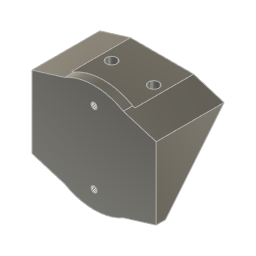
mount (Autodesk Fusion 360 design; units mm, degrees)
Autodesk Fusion 360 part; units mm, degrees
sketch "Sketch1" plane through (0, 0, 0) normal (0, 1, 0) x (1, 0, 0)
  circle A0 centre (0, 0) radius 1.4
  circle A1 centre (0, -30.9) radius 1.4
  line L0 (0, -30.9) -> (0, 0) construction
  line L1 (-26.5, -15.45) -> (26.5, -15.45) construction
  line L2 (26.5, -0.05) -> (-26.5, -0.05)
  line L3 (-26.5, -0.05) -> (-26.5, -30.85)
  line L4 (-26.5, -30.85) -> (26.5, -30.85)
  line L5 (26.5, -30.85) -> (26.5, -0.05)
  line L6 (26.5, -0.05) -> (-26.5, -30.85) construction
  line L7 (-26.5, -0.05) -> (26.5, -30.85) construction
  line L8 (0, -38.45) -> (0, 7.55) construction
  line L9 (-26.5, -30.85) -> (-12.5, -35.15)
  line L10 (-12.5, -35.15) -> (0, -35.15)
  line L11 (26.5, -30.85) -> (12.5, -35.15)
  arc A2 (-12.5, -35.15) -> (12.5, -35.15) centre (0, -13.1258) ccw
  line L12 (-26.5, -0.05) -> (-12.5, 4.25)
  arc A3 (12.5, 4.25) -> (-12.5, 4.25) centre (0, -17.7742) ccw
  line L13 (26.5, -0.05) -> (12.5, 4.25)
  point P0 (0, -15.45)
  point P1 (0, -15.45)
  point P2 (0, -15.45)
  point P3 (0, -15.45)
  dimension "d1" = 2.8
  dimension "d2" = 2.8
  dimension "d3" = 30.9
  dimension "d4" = 53
  dimension "d5" = 53
  dimension "d6" = 30.8
  dimension "d7" = 14
  dimension "d8" = 19.7
  dimension "d9" = 46
  constraint coincident A0.centre L0.end
  constraint coincident A1.centre L0.start
  constraint vertical L0
  constraint horizontal L1
  constraint midpoint L1 P3
  constraint midpoint L0 P3
  constraint coincident P3 P2
  constraint horizontal L2
  constraint perpendicular L2 L3
  constraint parallel L2 L4
  constraint parallel L3 L5
  constraint coincident L6 P3
  constraint coincident L7 P3
  constraint perpendicular L1 L8
  constraint midpoint L8 P3
  constraint coincident L8 L10.end
  constraint perpendicular L8 L10
  constraint symmetric L3.end L8 L4.end
  constraint symmetric L8 L9.end L11.end
  constraint coincident L8.start A2
  constraint symmetric L1 L3.end L2.end
  constraint symmetric L1 L9.end L12.end
  constraint symmetric L1 L4.end L2.start
  constraint symmetric L1 L11.end A3.start
  constraint symmetric L1 A2 A3
  measures "d1" diameter of A1
  measures "d2" diameter of A0
  measures "d3" distance of A0.centre A1.centre
  measures "d4" distance of L1.start L1.end
  measures "d5" distance of L3.end L4.end
  measures "d6" distance of L2.end L3.end
  measures "d7" horizontal distance of L3.end L9.end
  measures "d8" distance of L1 L9.end
  measures "d9" distance of L8.start L8.end
extrude "Extrude1" add sketch "Sketch1" along normal blind 4
hole "Hole1" at (0, 0, 30.9) at (0, 0, 0) direction (0, 1, 0) diameter 2.529 end through all
thread "Thread1" "ISO Metric profile 3.0 M3x0.5 6H"
sketch "Sketch2" plane through (0, 4, 0) normal (0, 1, 0) x (-1, 0, 0)
  circle A0 centre (0, 30.9) radius 1.2645
  circle A1 centre (0, 0) radius 1.2645
  line L0 (-26.5, 30.85) -> (-26.5, 0.05)
  line L1 (-26.5, 0.05) -> (-12.5, -4.25)
  arc A2 (-12.5, -4.25) -> (12.5, -4.25) centre (0, 17.7742) ccw
  line L2 (12.5, -4.25) -> (26.5, 0.05)
  line L3 (26.5, 0.05) -> (26.5, 30.85)
  line L4 (26.5, 30.85) -> (12.5, 35.15)
  arc A3 (12.5, 35.15) -> (-12.5, 35.15) centre (0, 13.1258) ccw
  line L5 (-12.5, 35.15) -> (-26.5, 30.85)
  line L6 (-26.5, 30.85) -> (26.5, 30.85)
  line L7 (-26.5, 30.85) -> (26.5, 30.85)
  line L8 (26.5, 30.85) -> (26.5, 34.85)
  line L9 (26.5, 34.85) -> (-26.5, 34.85)
  line L10 (-26.5, 34.85) -> (-26.5, 30.85)
  circle A4 centre (0, 30.9) radius 2.5
  dimension "d20" = 4
  dimension "d21" = 5
  constraint horizontal L6
  constraint coincident L0.start L5.end
  constraint horizontal L7
  constraint vertical L8
  constraint horizontal L9
  constraint vertical L10
  constraint concentric A0 A4
  measures "d20" distance of L0.start L9.end
  measures "d21" diameter of A4
extrude "Extrude2" add sketch "Sketch2" along normal blind 25 contours L4 L5 L6 L7 L9 A4
sketch "Sketch3" plane through (0, 0, 30.85) normal (0, 0, -1) x (1, 0, 0)
  line L0 (26.5, -4) -> (-26.5, -4)
  line L1 (-26.5, -4) -> (-26.5, -29)
  line L2 (-26.5, -29) -> (26.5, -29)
  line L3 (26.5, -29) -> (26.5, -4)
  line L4 (-26.5, -16.5) -> (26.5, -16.5)
  line L5 (-9, -16.5) -> (-9, -29)
  line L6 (9, -16.5) -> (9, -29)
  line L7 (26.5, -4) -> (2.4995, -4)
  line L8 (2.4995, -29) -> (26.5, -29)
  line L9 (26.5, -29) -> (26.5, -4)
  line L10 (2.4995, -4) -> (2.4995, -29)
  dimension "d18" = 17.5
  dimension "d19" = 17.5
  constraint midpoint L1 L4.start
  constraint midpoint L3 L4.end
  constraint coincident L4 L5.start
  constraint coincident L2 L5.end
  constraint perpendicular L2 L5
  constraint coincident L4 L6.start
  constraint coincident L2 L6.end
  constraint perpendicular L2 L6
  measures "d18" distance of L1 L5
  measures "d19" distance of L3 L6
hole "Hole2" at (-9, 16.5, 30.85) at (9, 16.5, 30.85) direction (0, 0, 1) diameter 4.5 depth 4 tip angle 118
sketch "Sketch4" plane through (-26.5, 0, 0) normal (-1, 0, 0) x (0, -1, 0)
  line L0 (0, 0.05) -> (0, 30.85)
  line L1 (0, 30.85) -> (-4, 30.85)
  line L2 (-4, 30.85) -> (-4, 0.05)
  line L3 (-4, 0.05) -> (0, 0.05)
  line L4 (0, 30.85) -> (0, 35.15)
  line L5 (0, 35.15) -> (-4, 35.15)
  line L6 (-4, 35.15) -> (-4, 34.85)
  line L7 (-4, 34.85) -> (-29, 34.85)
  line L8 (-29, 34.85) -> (-29, 30.85)
  line L9 (-29, 30.85) -> (-4, 30.85)
  line L10 (-4, 30.85) -> (0, 30.85)
  line L11 (-29, 30.85) -> (-4, 0.05)
  constraint coincident L8.end L9.start
  constraint coincident L2.end L3.start
sketch "Sketch5" plane through (26.5, 0, 0) normal (1, 0, 0) x (0, 1, 0)
  line L0 (0, 30.85) -> (0, 0.05)
  line L1 (0, 0.05) -> (4, 0.05)
  line L2 (4, 0.05) -> (4, 30.85)
  line L3 (4, 30.85) -> (0, 30.85)
  line L4 (0, 35.15) -> (0, 30.85)
  line L5 (0, 30.85) -> (4, 30.85)
  line L6 (4, 30.85) -> (29, 30.85)
  line L7 (29, 30.85) -> (29, 34.85)
  line L8 (29, 34.85) -> (4, 34.85)
  line L9 (4, 34.85) -> (4, 35.15)
  line L10 (4, 35.15) -> (0, 35.15)
  line L11 (29, 30.85) -> (4, 0.05)
extrude "Extrude3" add sketch "Sketch5" against normal blind 4 contours L2 L6 L11
extrude "Extrude4" add sketch "Sketch4" against normal blind 4 contours L2 L9 L11
equation "d8 = ( 39.4 / 2 ) * 1 mm"
named bodies: "meterback"
